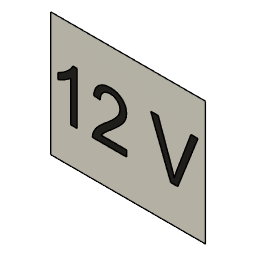
12_volt_label (Autodesk Fusion 360 design; units mm, degrees)
part number: 2025-04-13-10-20-13-952
Autodesk Fusion 360 part; units mm, degrees
sketch "Sticker" plane through (0, 0, 0) normal (0, 1, 0) x (1, 0, 0)
  line L0 (0, 0) -> (15, 0)
  line L1 (15, 0) -> (15, -12)
  line L2 (15, -12) -> (0, -12)
  line L3 (0, -12) -> (0, 0)
  dimension "d1" = 12
  dimension "d2" = 15
  constraint horizontal L0
  constraint vertical L1
  constraint horizontal L2
  constraint vertical L3
  constraint coincident L0.start L3.end
  measures "d1" distance of L0.end L1.end
  measures "d2" distance of L0.start L0.end
extrude "Extrude1" add sketch "Sticker" along normal blind 0.01 makes body 1
sketch "Text" plane through (0, 0, 0) normal (0, -1, 0) x (1, 0, 0)
  line L0 (15, 12) -> (0, 12)
  line L1 (0, 12) -> (0, 0)
  line L2 (0, 0) -> (15, 0)
  line L3 (15, 0) -> (15, 12)
  line L4 (0, 0) -> (15, 0) construction
  line L5 (15, 0) -> (15, 12) construction
  line L6 (15, 12) -> (0, 12) construction
  line L7 (0, 12) -> (0, 0) construction
  dimension "d5" = 5
  dimension "d8" = 0
  text T0 "12 V" font "Arial" height 5 align centre middle in box 15 x 12 at (0, 0) x (1, 0) y (0, 1) spacing 1 kerned
  constraint coincident L2.end
  constraint coincident L0.end
extrude "Extrude2" add sketch "Text" along normal blind 0.01 separate body text T0 makes body 2 at (5.4445, 0, 3.6967) makes body 3 at (10.6139, 0, 7.2892) makes body 4 at (2.3602, 0, 6.4775)
equation "d8 = 12 V"
named bodies: "Sticker", "Text 2", "Text 3", "Text 1"
